Ofengriff_Blocker_v1 (Autodesk Fusion 360 design; units mm, degrees)
Autodesk Fusion 360 part; units mm, degrees
note: some values were not read from the file. Set by a fixed rule: which sketch regions a step uses; which face or edge a step refers to.
sketch "Sketch1" plane through (0, 0, 0) normal (0, 1, 0) x (1, 0, 0)
  line L0 (0, 0) -> (0, -42)
  circle A0 centre (-0.0004, -49) radius 7
  line L1 (0, 0) -> (25.5, 0)
  line L2 (0, 0) -> (-25.5, 0)
  circle A1 centre (-0.0004, -49) radius 11
  line L3 (25.5, 0) -> (25.5, 7)
  line L4 (25.5, 7) -> (30.0218, 7)
  line L5 (30.0218, 7) -> (30.0218, -0.0156)
  line L6 (30.0218, -0.0156) -> (10.3053, -52.8461)
  line L7 (-25.5, 0) -> (-10.574, -52.0331)
  line L8 (-0.0004, -49) -> (-0.0004, -54)
  line L9 (-13, -65) -> (14, -65)
  line L10 (14, -65) -> (14, -54)
  line L11 (14, -54) -> (-13, -54)
  line L12 (-13, -54) -> (-13, -65)
  dimension "d1" = 42
  dimension "d2" = 14
  dimension "d3" = 25.5
  dimension "d4" = 22
  dimension "d5" = 7
  constraint coincident L0.start L1.start
  constraint vertical L0
  constraint coincident L0.end A0
  constraint perpendicular L0 L1
  constraint perpendicular L0 L2
  constraint equal L1 L2
  constraint concentric A0 A1
  constraint perpendicular L1 L3
  constraint perpendicular L3 L4
  constraint perpendicular L4 L5
  constraint coincident A1 L6.end
  constraint tangent A1 L6
  constraint coincident A1 L7.end
  constraint tangent A1 L7
  constraint coincident A0.centre A1.centre
  constraint vertical L8
  constraint horizontal L9
  constraint vertical L10
  constraint horizontal L11
  constraint vertical L12
  measures "d1" distance of L0.start L0.end
  measures "d2" diameter of A0
  measures "d3" distance of L0.start L1.end
  measures "d4" diameter of A1
  measures "d5" distance of L1.end L3.end
extrude "Extrude1" add sketch "Sketch1" along normal blind 50 contours L0 L1 A1 L3 L4 L5 L6 | L0 L2 A1 L7 | L0 A0 A1 L11 | L0 A0 A1 L11
fillet "Fillet1" radius 1 13 faces at (-6.5324, 16.6667, 54) (8.1645, 16.6667, 54) (-8.5, 33.3333, 0) (27.0073, 16.6667, -7) (9.8604, 16.6667, 53.8748) (23.4496, 33.3333, 17.6258) (30.0218, 16.6667, -4.6615) (-9.9031, 33.3333, 53.7893) (-20.5247, 16.6667, 17.3444) (25.5, 16.6667, -2.3333) (-7.0003, 33.3333, 49.0475) (-9.5017, 50, 14.2259) (-9.5017, 0, 14.2259)
